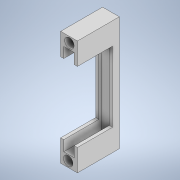
# Autodesk Inventor part: Stand Lower covet
Saved by Autodesk Inventor 2022 (Build 260153000, 153)
## iProperties
Created: 2022-08-22
Part Number: Stand Lower covet
Material: Generic
Document SubType Name: Modeling
Designer: yashm
Density: 1 g/cm^3
Appearance: Default
Author: yashm
Autodesk Inventor part; units mm, degrees
ref_plane "YZ Plane" through (0, 0, 0) normal (1, 0, 0) x (0, 1, 0)
ref_plane "XZ Plane" through (0, 0, 0) normal (0, 1, 0) x (-1, 0, 0)
ref_plane "XY Plane" through (0, 0, 0) normal (0, 0, 1) x (1, 0, 0)
sketch "Sketch1" plane through (0, 0, 0) normal (0, 0, 1) x (1, 0, 0)
  line L0 (0, 0) -> (8, 0)
  line L1 (8, 0) -> (8, 50.5)
  line L2 (8, 50.5) -> (0, 50.5)
  line L3 (0, 50.5) -> (0, 0)
  dimension "d0" = 8
  dimension "d1" = 50.5
  constraints: 8 end point, 2 parallel, 1 horizontal, 1 perpendicular
  measures "d0" distance of L1.end L2.end
  measures "d1" distance of L2.end L0.start
extrude "Extrusion1" add sketch "Sketch1" along normal blind 20
sketch "Sketch2" plane through (0, 0, 20) normal (0, 0, 1) x (1, 0, 0)
  line L0 (8, 0) -> (8, 50.5) projected
  line L1 (0, 42) -> (8, 42)
  line L2 (8, 42) -> (8, 8.5)
  line L3 (8, 8.5) -> (0, 8.5)
  line L4 (0, 8.5) -> (0, 42)
  line L5 (8, 50.5) -> (0, 50.5) projected
  line L6 (0, 0) -> (8, 0) projected
  dimension "d4" = 33.5
  dimension "d5" = 8.5
  dimension "d6" = 8.5
  constraints: 8 end point, 2 parallel, 1 horizontal, 1 perpendicular, 1 point on line
  measures "d4" distance of L3.end L1.start
  measures "d5" distance between parallel lines of L5 L1
  measures "d6" distance between parallel lines of L6 L3
extrude "Extrusion2" cut sketch "Sketch2" against normal blind 16.74
sketch "Sketch3" plane through (0, 0, 20) normal (0, 0, 1) x (1, 0, 0)
  line L0 (1.5, 47) -> (6.5, 47)
  line L1 (6.5, 47) -> (6.5, 3.5)
  line L2 (6.5, 3.5) -> (1.5, 3.5)
  line L3 (1.5, 3.5) -> (1.5, 47)
  line L4 (0, 50.5) -> (0, 42) projected
  line L5 (0, 42) -> (8, 42) projected
  line L6 (8, 8.5) -> (0, 8.5) projected
  point P0 (0, 0)
  dimension "d9" = 5
  dimension "d10" = 1.5
  dimension "d11" = 5
  dimension "d12" = 5
  constraints: 8 end point, 2 parallel, 1 horizontal, 1 perpendicular
  measures "d9" distance of L0.start L0.end
  measures "d10" distance between parallel lines of L4 L3
  measures "d11" distance between parallel lines of L0 L5
  measures "d12" distance between parallel lines of L6 L2
extrude "Extrusion3" cut sketch "Sketch3" against normal blind 17.75
sketch "Sketch4" plane through (0, 0, 20) normal (0, 0, 1) x (1, 0, 0)
  line L0 (8, 50.5) -> (0, 50.5) projected
  line L1 (0, 50.5) -> (8, 50.5)
  line L2 (8, 50.5) -> (8, 52.5)
  line L3 (8, 52.5) -> (0, 52.5)
  line L4 (0, 52.5) -> (0, 50.5)
  line L5 (0, 0) -> (8, 0) projected
  line L6 (0, 0) -> (8, 0)
  line L7 (8, 0) -> (8, -2)
  line L8 (8, -2) -> (0, -2)
  line L9 (0, -2) -> (0, 0)
  dimension "d15" = 2
  constraints: 16 end point, 4 parallel, 2 horizontal, 2 perpendicular, 1 collinear, 1 point on line
  measures "d15" distance of L1.end L2.end
extrude "Extrusion4" add sketch "Sketch4" against normal up to surface (20 mm away)
sketch "Sketch5" plane through (0, 0, 20) normal (0, 0, 1) x (1, 0, 0)
  circle A0 centre (4.1899, 49.75) radius 2.25
  circle A1 centre (3.6194, 0.75) radius 2.25
  line L0 (0, -2) -> (8, -2) projected
  line L1 (6.5, 3.5) -> (1.5, 3.5) projected
  line L2 (1.5, 47) -> (6.5, 47) projected
  point P0 (0, 0)
  dimension "d18" = 5.5
  dimension "d19" = 4.5
  dimension "d20" = 2.75
  dimension "d21" = 2.75
  constraints: 2 centre point, 1 equal radius
  measures "d18" distance between parallel lines of L0 L1
  measures "d19" diameter of A1
  measures "d20" distance from line of L1 A1.centre
  measures "d21" distance from line of L2 A0.centre
extrude "Extrusion5" cut sketch "Sketch5" against normal up to surface (20 mm away)
body "Solid1"
